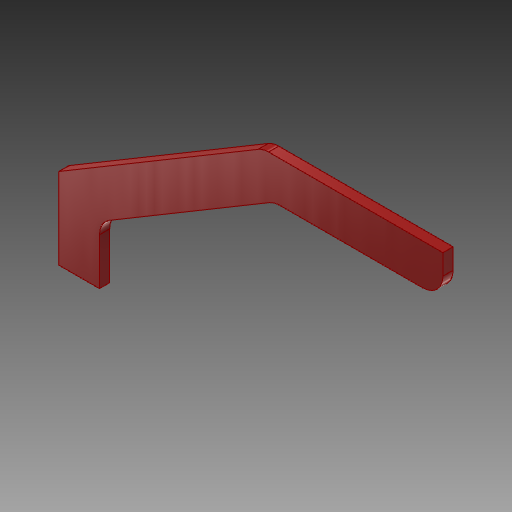
# Autodesk Inventor part: XZ chain Support
Saved by Autodesk Inventor 2019 (Build 230136000, 136)
## iProperties
Created: 2018-01-22
Part Number: XZ chain Support
Material: Steel
Document SubType Name: Modeling
Designer: torba
Density: 7.85 g/cm^3
Appearance: Red
Author: torba
Autodesk Inventor part; units mm, degrees
ref_plane "YZ Plane" through (0, 0, 0) normal (1, 0, 0) x (0, 1, 0)
ref_plane "XZ Plane" through (0, 0, 0) normal (0, 1, 0) x (-1, 0, 0)
ref_plane "XY Plane" through (0, 0, 0) normal (0, 0, 1) x (1, 0, 0)
sketch "Sketch1" plane through (0, 0, 0) normal (1, 0, 0) x (0, 1, 0)
  line L0 (166.3556, -22.225) -> (191.7556, -22.225)
  line L1 (166.3556, -22.225) -> (166.3556, -58.5973)
  line L2 (191.7556, -22.225) -> (191.7556, -73.025)
  line L3 (-48.7444, -149.225) -> (-48.7444, -123.825)
  line L4 (-48.7444, -123.825) -> (56.958, -123.825)
  line L5 (56.958, -123.825) -> (166.3556, -58.5973)
  line L6 (191.7556, -73.025) -> (63.9556, -149.225)
  line L7 (63.9556, -149.225) -> (-48.7444, -149.225)
  point P0 (0, 0)
  dimension "d96" = 50.8
  dimension "d97" = 25.4
  constraints: 16 end point, 3 vertical, 2 horizontal, 1 perpendicular
  measures "d96" distance of L0.end L2.end
  measures "d97" distance of L3.start L3.end
extrude "Extrusion2" add sketch "Sketch1" along normal blind 6.35
fillet "Fillet1" radius 12.7 1 edges at (3.175, -48.7444, -123.825)
fillet "Fillet2" radius 12.7 3 edges at (3.175, 56.958, -123.825) (3.175, 166.3556, -58.5973) (3.175, 63.9556, -149.225)
body "Solid2"
